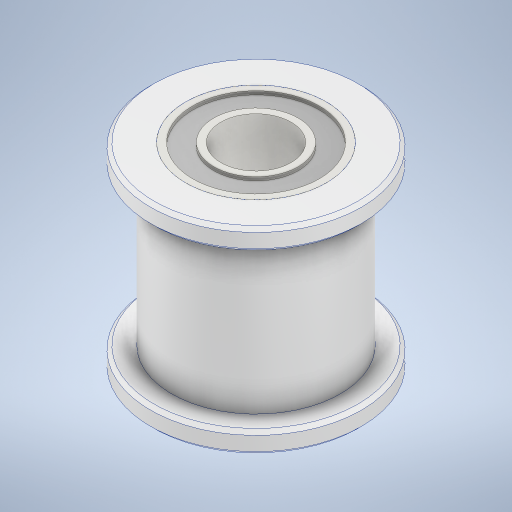
# Autodesk Inventor part: 10mm 20T Smooth Idler Pulley 5mm Bore
Saved by Autodesk Inventor 2024 (Build 280153000, 153)
## iProperties
Created: 2023-06-15
Part Number: 10mm 20T Smooth Idler Pulley 5mm Bore
Material: Aluminum 6061
Document SubType Name: Modeling
Designer: Ishaan
Density: 2.7 g/cm^3
Appearance: Aluminum - Flat
Author: Ishaan
Autodesk Inventor part; units mm, degrees
ref_plane "YZ Plane" through (0, 0, 0) normal (1, 0, 0) x (0, 1, 0)
sketch "Sketch1" plane through (0, 0, 0) normal (0, 0, 1) x (1, 0, 0)
  line L0 (0, 0) -> (-7.5, 0)
  line L1 (-7.5, 0) -> (-7.5, 1.5)
  line L2 (-7.5, 1.5) -> (0, 1.5)
  line L3 (0, 1.5) -> (0, 0)
  line L4 (0, 1.5) -> (-6, 1.5)
  line L5 (-6, 1.5) -> (-6, 12.5)
  line L6 (-6, 12.5) -> (0, 12.5)
  line L7 (0, 12.5) -> (0, 1.5)
  line L8 (0, 12.5) -> (-7.5, 12.5)
  line L9 (-7.5, 12.5) -> (-7.5, 14)
  line L10 (-7.5, 14) -> (0, 14)
  line L11 (0, 14) -> (0, 12.5)
  line L12 (0, 14) -> (-5, 14)
  line L13 (-5, 14) -> (-5, 0)
  line L14 (-5, 0) -> (0, 0)
  line L15 (0, 0) -> (0, 14)
  point P0 (-5, 14)
  point P1 (-6, 1.5)
  dimension "d0" = 7.5
  dimension "d1" = 5
  dimension "d2" = 14
  dimension "d3" = 11
  dimension "d4" = 1.5
  dimension "d5" = 6
  constraints: 32 end point, 8 parallel, 4 horizontal, 4 perpendicular, 2 point on line
  measures "d0" distance between parallel lines of L3 L1
  measures "d1" distance between parallel lines of L13 L3
  measures "d2" distance between parallel lines of L0 L10
  measures "d3" distance between parallel lines of L2 L8
  measures "d4" distance between parallel lines of L0 L2
  measures "d5" distance between parallel lines of L7 L5
revolve "Revolution1" add sketch "Sketch1" angle 360 about axis through (0, 0, 0) along (0, 1, 0) contours L0 L1 L2 L13 | L2 L5 L6 L13 | L6 L8 L9 L10 L13
chamfer "Chamfer2" distance 0.25 angle 45 4 edges at (7.5, 12.5, 0) (7.5, 1.5, 0) (7.5, 0, 0) (7.5, 14, 0)
ref_plane "Work Plane5" through (0, 12, 0) normal (0, 1, 0) x (1, 0, 0)
sketch "Sketch6" plane through (0, 12, 0) normal (0, 1, 0) x (1, 0, 0)
  circle A0 centre (0, 0) radius 5
  circle A1 centre (0, 0) radius 2.5
  circle A2 centre (0, 0) radius 4.5
  circle A3 centre (0, 0) radius 3
  dimension "d36" = 10
  dimension "d37" = 5
  dimension "d38" = 0.5
  dimension "d39" = 0.5
  constraints: 4 centre point, 2 coincident
  measures "d36" diameter of A0
  measures "d37" diameter of A1
  measures "d38" radial gap between concentric circles of A0 A2
  measures "d39" radial gap between concentric circles of A1 A3
extrude "Extrusion3" add sketch "Sketch6" along normal mid plane 4 separate body
extrude "Extrusion4" add sketch "Sketch6" along normal mid plane 3.5 contours A2 bodies 2
ref_plane "Work Plane4" through (0, 7, 0) normal (0, -1, 0) x (1, 0, 0)
mirror "Mirror3" about plane through (0, 7, 0) normal (0, -1, 0) bodies 2
body "Solid1"
